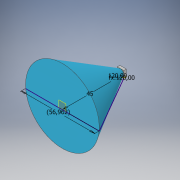
# Autodesk Inventor part: led 5050
Saved by Autodesk Inventor 2019 (Build 230136000, 136)
## iProperties
Created: 2021-08-02
Part Number: led 5050
Material: Generic
Document SubType Name: Modeling
Designer: Lix
Density: 1 g/cm^3
Appearance: Default
Author: Lix
Autodesk Inventor part; units mm, degrees
ref_plane "YZ Plane" through (0, 0, 0) normal (1, 0, 0) x (0, 1, 0)
ref_plane "XZ Plane" through (0, 0, 0) normal (0, 1, 0) x (-1, 0, 0)
ref_plane "XY Plane" through (0, 0, 0) normal (0, 0, 1) x (1, 0, 0)
sketch "Sketch1" plane through (0, 0, 0) normal (0, 0, 1) x (1, 0, 0)
  line L0 (-2.5, 2.5) -> (2.5, 2.5)
  line L1 (2.5, 2.5) -> (2.5, -2.5)
  line L2 (2.5, -2.5) -> (-2.5, -2.5)
  line L3 (-2.5, -2.5) -> (-2.5, 2.5)
  line L4 (-2.5, 2.5) -> (2.5, -2.5) construction
  line L5 (2.5, 2.5) -> (-2.5, -2.5) construction
  circle A0 centre (0, 0) radius 2.25
  dimension "d0" = 5
  dimension "d1" = 5
  dimension "d2" = 4.5
  constraints: 12 end point, 2 midpoint, 2 parallel, 1 centre point, 1 coincident, 1 horizontal, 1 perpendicular
  measures "d0" distance of L1.end L2.end
  measures "d1" distance of L0.end L1.end
  measures "d2" diameter of A0
extrude "Extrusion1" add sketch "Sketch1" along normal blind 2 contours L0 L1 L2 L3 | A0
sketch "Sketch2" plane through (-2.5, -2.5, 0) normal (0, -1, 0) x (1, 0, 0)
  line L0 (5, 0) -> (0, 0) projected
  line L1 (5, 0) -> (5, 2) projected
  line L2 (0, 2) -> (5, 2) projected
  line L3 (0, 0) -> (0, 2) projected
  line L4 (5, 2) -> (0, 2) projected
  line L5 (0, 2) -> (-25.9808, 47)
  line L6 (-25.9808, 47) -> (30.9808, 47)
  line L7 (5, 2) -> (30.9808, 47)
  point P0 (2.5, 0)
  dimension "d5" = 120
  dimension "d6" = 120
  dimension "d7" = 45
  dimension "d9" = 56.9615
  constraints: 6 end point, 1 parallel
  measures "d5" angle of L2 L5
  measures "d6" angle of L7 L2
  measures "d7" distance between parallel lines of L6 L2
  measures "d9" distance of L5.end L6.end
sketch "Sketch3" plane through (0, 0, 2) normal (0, 0, 1) x (1, 0, 0)
  circle A0 centre (0, 0) radius 2.5
  constraints: 1 centre point, 1 coincident
ref_plane "Work Plane1" through (0, 0, 47) normal (0, 0, 1) x (1, 0, 0)
sketch "Sketch4" plane through (0, 0, 47) normal (0, 0, 1) x (1, 0, 0)
  circle A0 centre (0, 0) radius 28.5
  point P0 (28.4808, -2.5)
  dimension "d10" = 57
  constraints: 1 centre point, 1 coincident
  measures "d10" diameter of A0
loft "Loft1" add profiles "Sketch3", "Sketch4"
equation "\"d6\" = d5"
body "Solid1"
